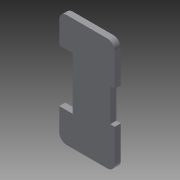
# Autodesk Inventor part: Base
Saved by Autodesk Inventor 2015 (Build 190159000, 159)
## iProperties
Created: 2016-06-05
Part Number: Base
Material: Generic
Document SubType Name: Modeling
Designer: EriveltonDell
Density: 1 g/cm^3
Appearance: Default
Author: EriveltonDell
Autodesk Inventor part; units mm, degrees
ref_plane "YZ Plane" through (0, 0, 0) normal (1, 0, 0) x (0, 1, 0)
ref_plane "XZ Plane" through (0, 0, 0) normal (0, 1, 0) x (-1, 0, 0)
ref_plane "XY Plane" through (0, 0, 0) normal (0, 0, 1) x (1, 0, 0)
sketch "Sketch1" plane through (0, 0, 0) normal (0, 1, 0) x (-1, 0, 0)
  line L0 (10, 0) -> (64, 0)
  line L1 (64, 150) -> (10, 150)
  line L2 (0, 10) -> (0, 53)
  line L3 (0, 53) -> (6, 53)
  line L4 (6, 53) -> (6, 97)
  line L5 (6, 97) -> (0, 97)
  line L6 (74, 10) -> (74, 40)
  line L7 (74, 40) -> (56, 40)
  line L8 (56, 40) -> (56, 110)
  line L9 (56, 110) -> (74, 110)
  line L10 (74, 0) -> (74, 40)
  line L11 (74, 110) -> (74, 140)
  line L12 (0, 140) -> (0, 97)
  line L13 (0, 53) -> (0, 0)
  arc A0 (74, 140) -> (64, 150) centre (64, 140) ccw
  arc A1 (10, 150) -> (0, 140) centre (10, 140) ccw
  arc A2 (0, 10) -> (10, 0) centre (10, 10) ccw
  arc A3 (64, 0) -> (74, 10) centre (64, 10) ccw
  point P0 (74, 150)
  point P1 (0, 150)
  dimension "d0" = 74
  dimension "d1" = 150
  dimension "d2" = 53
  dimension "d3" = 6
  dimension "d4" = 44
  dimension "d5" = 40
  dimension "d6" = 18
  dimension "d7" = 70
  dimension "d8" = 10
  constraints: 28 end point, 10 perpendicular, 8 point on circle, 8 point on line, 8 tangent, 5 parallel, 4 centre point, 3 equal radius, 1 horizontal
  measures "d0" distance of point (0, 150) point (74, 150)
  measures "d1" distance of point (74, 150) L10.start
  measures "d2" distance of L13.end L2.end
  measures "d3" distance of L2.end L3.end
  measures "d4" distance of L3.end L4.end
  measures "d5" distance of L10.start L6.end
  measures "d6" distance of L6.end L7.end
  measures "d7" distance of L7.end L8.end
  measures "d8" radius of A0
extrude "Extrusion1" add sketch "Sketch1" along normal blind 8
body "Solid1"
